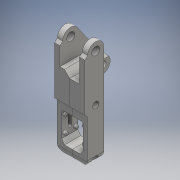
# Autodesk Inventor part: Arm - effector base
Saved by Autodesk Inventor 2016 (Build 200138000, 138)
## iProperties
Created: 2016-04-30
Part Number: Arm - effector base
Material: Generic
Document SubType Name: Modeling
Designer: Ali
Density: 1 g/cm^3
Appearance: Default
Author: Ali
Autodesk Inventor part; units mm, degrees
ref_plane "YZ Plane" through (0, 0, 0) normal (1, 0, 0) x (0, 1, 0)
ref_plane "XZ Plane" through (0, 0, 0) normal (0, 1, 0) x (-1, 0, 0)
sketch "Sketch8" plane through (0, 0, 0) normal (1, 0, 0) x (0, 1, 0)
  circle A0 centre (0, 0) radius 4.5
  circle A1 centre (24.3, -34.6) radius 4.5
  arc A2 (7.3651, 5.1726) -> (-9, 0) centre (0, 0) ccw
  arc A3 (24.3, -43.6) -> (31.6651, -29.4274) centre (24.3, -34.6) ccw
  line L0 (7.3651, 5.1726) -> (31.6651, -29.4274)
  line L1 (24.3, -43.6) -> (9, -43.6)
  line L2 (9, -43.6) -> (9, -103.6)
  line L3 (9, -103.6) -> (-9, -103.6)
  line L4 (-9, -103.6) -> (-9, 0)
  arc A4 (-9, -103.6) -> (9, -103.6) centre (0, -103.6) ccw
  dimension "d64" = 9
  dimension "d65" = 9
  dimension "d66" = 34.6
  dimension "d67" = 24.3
  dimension "d68" = 18
  dimension "d69" = 18
  dimension "d70" = 60
  dimension "d71" = 18
  constraints: 10 end point, 6 point on circle, 5 centre point, 5 tangent, 3 coincident, 1 horizontal, 1 perpendicular, 1 vertical
  measures "d64" diameter of A0
  measures "d65" diameter of A1
  measures "d66" vertical distance of A1.centre point (0, 0)
  measures "d67" horizontal distance of point (0, 0) A1.centre
  measures "d68" diameter of A2
  measures "d69" diameter of A3
  measures "d70" distance of L1.end L2.end
  measures "d71" distance of L2.end L3.end
extrude "Extrusion8" add sketch "Sketch8" along normal blind 6
sketch "Sketch9" plane through (6, 0, 0) normal (1, 0, 0) x (0, 0, -1)
  circle A0 centre (34.6, 24.3) radius 4.5 projected
  line L0 (0, -9) -> (63.6, -9)
  line L1 (43.6, 9) -> (43.6, 24.3) projected
  arc A1 (43.6, 24.3) -> (29.4274, 31.6651) centre (34.6, 24.3) ccw projected
  line L2 (29.4274, 31.6651) -> (-5.1726, 7.3651) projected
  line L3 (23.3108, 9) -> (23.3108, -9)
  line L4 (23.3108, -9) -> (43.6, -9)
  line L5 (43.6, 9) -> (63.6, 9)
  line L6 (63.6, 9) -> (63.6, -9)
  line L7 (63.6, -9) -> (43.6, -9)
  line L8 (23.3108, 9) -> (23.3108, 27.3693)
  line L9 (99.6, 9) -> (99.6, -9)
  line L10 (99.6, 9) -> (63.6, 9)
  line L11 (63.6, 9) -> (43.6, 9)
  line L12 (63.6, -9) -> (99.6, -9)
  arc A2 (103.6, -9) -> (103.6, 9) centre (103.6, 0) ccw projected
  line L13 (99.6, 9) -> (103.6, 9)
  line L14 (103.6, 9) -> (43.6, 9) projected
  line L15 (103.6, -9) -> (99.6, -9)
  line L16 (0, -9) -> (103.6, -9) projected
  point P0 (14.6712, 21.3016)
  dimension "d74" = 20
  dimension "d80" = 36
  constraints: 26 end point, 3 perpendicular, 3 point on line, 2 collinear, 2 point on circle, 1 horizontal, 1 parallel, 1 vertical
  measures "d74" distance of L0.end L7.end
  measures "d80" distance between parallel lines of L9 L6
extrude "Extrusion9" add sketch "Sketch9" along normal blind 11 contours L3 L8 L2 A1 L1 L5 L6 L0 | L9 L13 A2 L15
chamfer "Chamfer4" distance 6 angle 45 1 edges at (17, 9.1846, -23.3108)
sketch "Sketch10" plane through (0, 9, -43.6) normal (0, 1, 0) x (1, 0, 0)
  line L0 (0, 60) -> (17, 60) projected
  line L1 (17, 60) -> (17, 69) projected
  arc A0 (17, 69) -> (0, 60.9642) centre (17, 47) ccw
  line L2 (0, 60) -> (0, 60.9642)
  line L3 (0, 60) -> (0, 69) projected
  line L4 (0, 60) -> (29.3346, 60)
  line L5 (29.3346, 60) -> (29.3346, -58.462)
  line L6 (29.3346, -58.462) -> (0, -58.462)
  line L7 (0, -58.462) -> (0, 60)
  point P0 (17, 56)
  dimension "d81" = 9
  constraints: 10 end point, 2 parallel, 2 point on circle, 1 centre point, 1 coincident, 1 horizontal, 1 perpendicular, 1 point on line
  measures "d81" distance of point (17, 56) point (17, 47)
extrude "Extrusion10" cut sketch "Sketch10" along normal through all both and the other way through all keep common part
fillet "Fillet1" radius 6.5 1 edges at (0, 0, -104.5642)
sketch "Sketch11" plane through (6, 0, 0) normal (1, 0, 0) x (0, 0, -1)
  line L0 (63.6, 9) -> (63.6, -9) projected
  line L1 (63.6, -9) -> (99.6, -9) projected
  line L2 (99.6, -9) -> (99.6, 9) projected
  line L3 (99.6, 9) -> (63.6, 9) projected
  point P0 (0, 0)
extrude "Extrusion11" cut sketch "Sketch11" against normal blind 1
sketch "Sketch12" plane through (5, 0, 0) normal (1, 0, 0) x (0, 0, -1)
  line L0 (63.6, -9) -> (63.6, 9) projected
  line L1 (63.6, 9) -> (99.6, 9) projected
  circle A0 centre (72.6, 6) radius 1.95
  circle A1 centre (90.6, 6) radius 1.95
  circle A2 centre (72.6, -6) radius 1.95
  circle A3 centre (90.6, -6) radius 1.95
  point P0 (0, 0)
  dimension "d87" = 3.9
  dimension "d90" = 18
  dimension "d93" = 12
  dimension "d96" = 3
  dimension "d97" = 9
  constraints: 4 centre point, 1 horizontal, 1 vertical, 6 other
  measures "d87" diameter of A0
  measures "d90" distance of A0.centre A1.centre
  measures "d93" distance of A0.centre A2.centre
  measures "d96" distance from line of L1 A0.centre
  measures "d97" distance from line of L0 A0.centre
extrude "Extrusion12" add sketch "Sketch12" along normal blind 3
chamfer "Chamfer5" distance 0.8 angle 45 4 edges at (8, 6, -70.65) (8, 6, -88.65) (8, -6, -88.65) (8, -6, -70.65)
sketch "Sketch13" plane through (5, 0, 0) normal (1, 0, 0) x (0, 0, -1)
  line L0 (63.6, -9) -> (63.6, 9) projected
  line L1 (76.4835, 0) -> (86.7165, 0) construction
  line L2 (76.4835, -2) -> (86.7165, -2)
  line L3 (86.7165, 2) -> (76.4835, 2)
  arc A0 (76.4835, 2) -> (76.4835, -2) centre (76.4835, 0) ccw
  arc A1 (86.7165, -2) -> (86.7165, 2) centre (86.7165, 0) ccw
  line L4 (63.6, -9) -> (63.6, 9) projected
  point P0 (0, 0)
  point P1 (81.6, 0)
  point P2 (63.6, 0)
  dimension "d103" = 4
  dimension "d104" = 18
  constraints: 8 end point, 4 point on circle, 4 tangent, 2 centre point, 2 midpoint, 1 horizontal, 1 parallel, 1 point on line
  measures "d103" diameter of A1
  measures "d104" distance from line of L0 point (81.6, 0)
extrude "Extrusion13" cut sketch "Sketch13" against normal through all
sketch "Sketch14" plane through (0, 0, 0) normal (-1, 0, 0) x (0, 0, 1)
  arc A0 (-76.4835, -2) -> (-76.4835, 2) centre (-76.4835, 0) ccw projected
  line L0 (-52.4835, 0) -> (-66.2095, 0) construction
  point P0 (-105.4194, 0)
  dimension "d107" = 24
  constraints: 2 end point, 2 point on line, 1 horizontal
  measures "d107" distance of A0.centre L0.start
hole "Hole3" at (0, 0, -52.4835) at (0, 0, -105.4194) direction (1, 0, 0) diameter 3.3 end through all counterbore diameter 7 counterbore depth 9
chamfer "Chamfer6" distance 1.85 angle 45 2 edges at (9, 0, -54.1335) (9, 0, -107.0694)
sketch "Sketch15" plane through (17, -9, -63.6) normal (0, 0, -1) x (-1, 0, 0)
  line L0 (0, 18) -> (12, 18) projected
  line L1 (0, 0) -> (0, 18) projected
  line L2 (12, 0) -> (0, 0) projected
  line L3 (12, 0) -> (12, 18) projected
  point P0 (17, 9)
extrude "Extrusion14" add sketch "Sketch15" along normal blind 3.5
chamfer "Chamfer7" distance 1.5 angle 45 1 edges at (5, 0, -67.1)
chamfer "Chamfer8" distance 3.25 distance2 4.5 1 edges at (5, 0, -99.6) measured on face at (9, 3, -99.6)
chamfer "Chamfer9" distance 3.5 angle 45 1 edges at (8.5, 9, -43.6)
ref_plane "Work Plane1" through (8.5, 0, 0) normal (-1, 0, 0) x (0, 0, 1)
sketch "Sketch16" plane through (8.5, 0, 0) normal (-1, 0, 0) x (0, 0, 1)
  circle A0 centre (-34.6, 24.3) radius 4.5 projected
  circle A1 centre (-34.6, 24.3) radius 3.5
  point P0 (0, 0)
  dimension "d129" = 1
  constraints: 1 centre point
  measures "d129" radial gap between concentric circles of A0 A1
extrude "Extrusion15" add sketch "Sketch16" along normal mid plane 9
chamfer "Chamfer10" distance 1 angle 45 2 edges at (4, 24.3, -38.1) (13, 24.3, -38.1)
sketch "Sketch17" plane through (0, -9, 0) normal (0, -1, 0) x (1, 0, 0)
  line L0 (17, -29.3108) -> (17, -67.1) projected
  line L1 (11, -23.3108) -> (17, -29.3108) projected
  line L2 (6, -23.3108) -> (11, -23.3108) projected
  line L3 (6, 0) -> (6, -23.3108) projected
  line L4 (0, 0) -> (6, 0) projected
  line L5 (0, 0) -> (0, -102.0018) projected
  line L6 (17, -59.623) -> (0, -59.623)
  line L7 (0, -102.0018) -> (0, -47.1) projected
  constraints: 2 end point, 2 point on line, 1 perpendicular
extrude "Extrusion16" add sketch "Sketch17" along normal blind 3
chamfer "Chamfer11" distance 3 angle 45 2 edges at (8.5, -12, -59.623) (3, -12, 0)
sketch "Sketch18" plane through (17, 0, 0) normal (1, 0, 0) x (0, 0, -1)
  line L0 (59.623, -9) -> (56.623, -12) projected
  line L1 (59.623, -9) -> (67.1, -9) projected
  line L2 (67.1, 9) -> (67.1, -9) projected
  line L3 (47.1, 9) -> (67.1, 9) projected
  line L4 (29.3108, 31.5832) -> (29.3108, -12) projected
  line L5 (56.623, -12) -> (29.3108, -12) projected
  circle A0 centre (52.4835, 0) radius 1.65 projected
  circle A1 centre (105.4194, 0) radius 1.65 projected
  arc A2 (103.6, -9) -> (112.6, 0) centre (103.6, 0) ccw projected
  arc A3 (112.6, 0) -> (103.6, 9) centre (103.6, 0) ccw projected
  line L6 (103.6, 9) -> (99.6, 9) projected
  line L7 (99.6, 9) -> (99.6, -9) projected
  line L8 (99.6, -9) -> (103.6, -9) projected
  line L9 (47.1, 9) -> (29.3108, 9)
  point P0 (0, 0)
  constraints: 2 end point, 1 perpendicular, 1 point on line
extrude "Extrusion17" add sketch "Sketch18" along normal blind 11 separate body contours L0 L5 L4 L9 L3 L2 L1 | A0 | A1 | L8 L7 L6 A3 A2
sketch "Sketch19" plane through (28, 0, 0) normal (1, 0, 0) x (0, 0, -1)
  line L0 (56.623, -12) -> (59.623, -9) projected
  line L1 (67.1, -9) -> (67.1, 9) projected
  line L2 (67.1, 9) -> (29.3108, 9) projected
  line L3 (29.3108, 9) -> (29.3108, -12) projected
  line L4 (29.3108, -12) -> (56.623, -12) projected
  arc A0 (103.6, -9) -> (103.6, 9) centre (103.6, 0) ccw projected
  line L5 (103.6, 9) -> (99.6, 9) projected
  line L6 (99.6, 9) -> (99.6, -9) projected
  line L7 (99.6, -9) -> (103.6, -9) projected
  line L8 (67.1, 9) -> (99.6, 9)
  line L9 (59.623, -9) -> (67.1, -9) projected
  line L10 (99.6, -9) -> (67.1, -9)
  arc A1 (-5.1726, 7.3651) -> (0, -9) centre (0, 0) ccw projected
  line L11 (3, -12) -> (0, -9) projected
  line L12 (23.3108, -12) -> (3, -12) projected
  line L13 (29.3108, -12) -> (23.3108, -12) projected
  line L14 (29.3108, 9) -> (0, 9)
  arc A2 (0, 9) -> (-5.1726, 7.3651) centre (0, 0) ccw
  circle A3 centre (0, 0) radius 4.5 projected
  constraints: 6 end point, 2 horizontal, 2 point on circle, 1 centre point, 1 coincident, 1 collinear
extrude "Extrusion18" add sketch "Sketch19" along normal blind 6 bodies 2
sketch "Sketch20" plane through (28, 0, 0) normal (-1, 0, 0) x (0, 0, 1)
  line L0 (-99.6, 9) -> (-99.6, -9) projected
  line L1 (-67.1, -9) -> (-99.6, -9) projected
  line L2 (-67.1, -9) -> (-67.1, 9) projected
  line L3 (-99.6, 9) -> (-67.1, 9) projected
  point P0 (0, 0)
extrude "Extrusion19" cut sketch "Sketch20" against normal blind 1 bodies 2
sketch "Sketch21" plane through (29, 0, 0) normal (-1, 0, 0) x (0, 0, 1)
  line L0 (-99.6, -9) -> (-99.6, 9) projected
  line L1 (-99.6, 9) -> (-67.1, 9) projected
  circle A0 centre (-90.6, 6) radius 1.95
  circle A1 centre (-72.6, 6) radius 1.95
  circle A2 centre (-90.6, -6) radius 1.95
  circle A3 centre (-72.6, -6) radius 1.95
  line L2 (-72.6, 6) -> (-72.6, -6) construction
  line L3 (-72.6, 0) -> (-94.0023, 0) construction
  point P0 (0, 0)
  dimension "d146" = 3.9
  dimension "d149" = 18
  dimension "d152" = 12
  dimension "d156" = 9
  dimension "d157" = 3
  constraints: 4 centre point, 4 end point, 2 horizontal, 2 vertical, 1 midpoint, 6 other
  measures "d146" diameter of A0
  measures "d149" distance of A0.centre L2.start
  measures "d152" distance of A0.centre A2.centre
  measures "d156" distance from line of L0 A0.centre
  measures "d157" distance from line of L1 L2.start
extrude "Extrusion20" add sketch "Sketch21" along normal blind 3 bodies 2
chamfer "Chamfer12" distance 0.8 angle 45 4 edges at (26, 6, -92.55) (26, 6, -74.55) (26, -6, -74.55) (26, -6, -92.55)
sketch "Sketch22" plane through (17, 9, -29.3108) normal (0, 1, 0) x (1, 0, 0)
  line L0 (0, 74.2892) -> (17, 74.2892) projected
  line L1 (0, 70.2892) -> (0, 74.2892) projected
  line L2 (21.4947, -41.8365) -> (0, -41.8365)
  line L3 (0, -41.8365) -> (0, 74.2892)
  line L4 (0, 74.2892) -> (21.4947, 74.2892)
  line L5 (21.4947, 74.2892) -> (21.4947, -41.8365)
  line L6 (0, 74.2892) -> (0, 83.2892) projected
  line L7 (17, 74.2892) -> (17, 75.2534)
  line L8 (17, 77.6086) -> (17, 74.6086) projected
  arc A0 (17, 75.2534) -> (0, 83.2892) centre (0, 61.2892) ccw
  point P0 (11, 74.2892)
  constraints: 10 end point, 2 parallel, 2 point on circle, 2 point on line, 1 centre point, 1 horizontal, 1 perpendicular
extrude "Extrusion21" cut sketch "Sketch22" against normal through all keep common part bodies 2
fillet "Fillet2" radius 6.5 1 edges at (34, 0, -104.5642)
sketch "Sketch23" plane through (34, 0, 0) normal (1, 0, 0) x (0, 0, -1)
  circle A0 centre (105.4194, 0) radius 1.65 projected
  circle A1 centre (52.4835, 0) radius 1.65 projected
hole "Hole4" at (34, 0, -52.4835) at (34, 0, -105.4194) direction (-1, 0, 0) diameter 3.3 end through all counterbore diameter 7 counterbore depth 9 bodies 2
sketch "Sketch24" plane through (25, 0, -52.4835) normal (1, 0, 0) x (0, 0, -1)
  circle A0 centre (0, 0) radius 3.5 projected
  circle A1 centre (0, 0) radius 1.65 projected
  circle A2 centre (52.9359, 0) radius 3.5 projected
  circle A3 centre (52.9359, 0) radius 1.65 projected
  line L0 (3.2909, 0) -> (1.6454, -2.85)
  line L1 (1.6454, -2.85) -> (-1.6454, -2.85)
  line L2 (-1.6454, -2.85) -> (-3.2909, 0)
  line L3 (-3.2909, 0) -> (-1.6454, 2.85)
  line L4 (-1.6454, 2.85) -> (1.6454, 2.85)
  line L5 (1.6454, 2.85) -> (3.2909, 0)
  line L6 (56.2268, 0) -> (54.5813, -2.85)
  line L7 (54.5813, -2.85) -> (51.2904, -2.85)
  line L8 (51.2904, -2.85) -> (49.645, 0)
  line L9 (49.645, 0) -> (51.2904, 2.85)
  line L10 (51.2904, 2.85) -> (54.5813, 2.85)
  line L11 (54.5813, 2.85) -> (56.2268, 0)
  point P0 (-52.4835, 0)
  dimension "d173" = 5.7
  dimension "d174" = 5.7
  constraints: 24 end point, 2 coincident, 26 other
  measures "d173" distance between parallel lines of L1 L4
  measures "d174" distance between parallel lines of L10 L7
extrude "Extrusion22" add sketch "Sketch24" along normal blind 2.5 contours A0 | A2 bodies 2
chamfer "Chamfer13" distance 0.64 angle 45 2 edges at (27.5, 0, -48.9835) (27.5, 0, -101.9194)
chamfer "Chamfer14" distance 1.5 angle 45 1 edges at (29, 0, -67.1)
chamfer "Chamfer15" distance 3.25 distance2 4.5 1 edges at (29, 0, -99.6) measured on face at (21, 3, -99.6)
